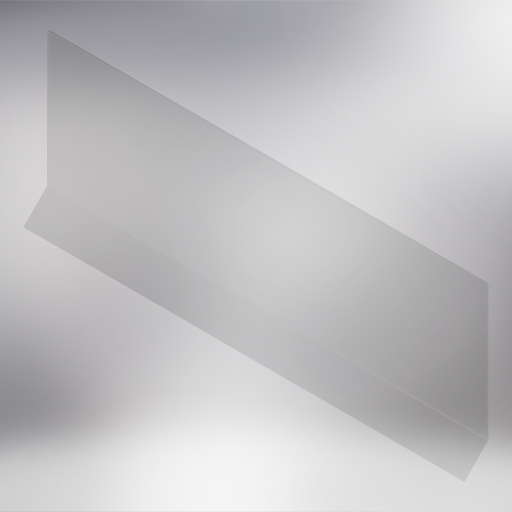
# Autodesk Inventor part: Wedge
Saved by Autodesk Inventor 2024 (Build 280153000, 153)
## iProperties
Created: 2023-12-18
Part Number: Wedge
Material: Polycarbonate, Clear
Document SubType Name: Modeling
Designer: aaron
Density: 1.2 g/cm^3
Appearance: Polycarbonate - Clear
Author: aaron
Autodesk Inventor part; units mm, degrees
ref_plane "YZ Plane" through (0, 0, 0) normal (1, 0, 0) x (0, 1, 0)
ref_plane "XZ Plane" through (0, 0, 0) normal (0, 1, 0) x (-1, 0, 0)
ref_plane "XY Plane" through (0, 0, 0) normal (0, 0, 1) x (1, 0, 0)
sketch "Sketch1" plane through (0, 0, 0) normal (1, 0, 0) x (0, 1, 0)
  line L0 (0, 0) -> (101.6, 0)
  line L1 (101.6, 0) -> (101.6, -1.5875)
  line L2 (101.6, -1.5875) -> (0, -1.5875)
  line L3 (0, -1.5875) -> (0, 0)
  circle A0 centre (0, -0.7937) radius 0.7937
  line L4 (0.5613, -0.2325) -> (-17.3992, 17.728)
  line L5 (-0.5613, -1.355) -> (-18.5218, 16.6055)
  line L6 (-17.3992, 17.728) -> (-18.5218, 16.6055)
  point P0 (0.3288, 0)
  dimension "d0" = 101.6
  dimension "d1" = 1.5875
  dimension "d2" = 25.4
  dimension "d3" = 135
  dimension "d4" = 25.4
  constraints: 14 end point, 3 parallel, 3 point on circle, 2 tangent, 1 centre point, 1 horizontal, 1 midpoint, 1 perpendicular
  measures "d0" distance of L1.end L2.end
  measures "d1" distance of L0.end L1.end
  measures "d2" distance of L4.start L4.end
  measures "d3" angle of L0 L4
  measures "d4" distance of L5.start L5.end
extrude "Extrusion1" add sketch "Sketch1" along normal blind 330.2
body "Solid1"
